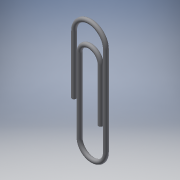
# Autodesk Inventor part: Paper Clip
Saved by Autodesk Inventor 2018 (Build 220112000, 112)
## iProperties
Created: 2005-07-15
Part Number: Paper Clip
Document SubType Name: Modeling
Designer: Administrator
Manufacturer: Standard
Standards Organization: Custom
Material: Generic
Density: 1 g/cm^3
Appearance: Default
Author: Administrator
Autodesk Inventor part; units mm, degrees
ref_plane "YZ Plane" through (0, 0, 0) normal (1, 0, 0) x (0, 1, 0)
ref_plane "XZ Plane" through (0, 0, 0) normal (0, 1, 0) x (-1, 0, 0)
sketch "Sketch1" plane through (0, 0, 0) normal (0, 0, 1) x (1, 0, 0)
  line L0 (-12.8211, -6.35) -> (-12.8211, 28.575)
  arc A0 (6.35, 28.575) -> (-12.8211, 28.575) centre (-3.2355, 28.575) ccw
  line L1 (6.35, 28.575) -> (6.35, -25.4)
  arc A1 (-9.525, -25.4) -> (6.35, -25.4) centre (-1.5875, -25.4) ccw
  line L2 (-9.525, -25.4) -> (-9.525, 19.05)
  arc A2 (3.175, 19.05) -> (-9.525, 19.05) centre (-3.175, 19.05) ccw
  line L3 (3.175, 19.05) -> (3.175, -12.7)
  constraints: 8 end point, 6 point on circle, 6 tangent, 3 centre point, 3 parallel, 1 vertical
ref_plane "Work Plane1" through (-12.8211, -6.35, 0) normal (0, 1, 0) x (-1, 0, 0)
sketch "Sketch2" plane through (-12.8211, -6.35, 0) normal (0, 1, 0) x (-1, 0, 0)
  circle A0 centre (0, 0) radius 1.27
  constraints: 1 centre point
sweep "Sweep1" add profiles "Sketch2" path "Sketch1"
body "Solid1"
